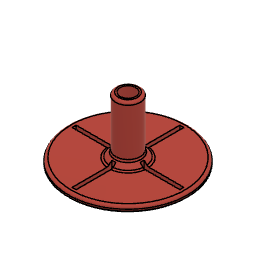
231213 drilling alignment tool 5.5 mm dia. v1 (Autodesk Fusion 360 design; units mm, degrees)
Autodesk Fusion 360 part; units mm, degrees
sketch "5.5 drilling alignment tool" plane through (0, 0, 0) normal (0, 1, 0) x (1, 0, 0)
  circle A0 centre (0, 0) radius 2.75
  circle A1 centre (0, 0) radius 4.35
  circle A2 centre (0, 0) radius 21
  line L0 (0, 0) -> (0, 30.5486) construction
  line L1 (0, 0) -> (37.4223, 0) construction
  line L2 (5, 0.7) -> (19, 0.7)
  line L3 (19, 0.7) -> (19, -0.7)
  line L4 (19, -0.7) -> (5, -0.7)
  line L5 (5, -0.7) -> (5, 0.7)
  dimension "d1" = 5.5
  dimension "d2" = 1.6
  dimension "d3" = 42
  dimension "d12" = 5
  dimension "d13" = 14
  dimension "d14" = 1.4
  constraint coincident A0.centre A1.centre
  constraint concentric A0 A2
  constraint vertical L0
  constraint perpendicular L0 L1
  constraint horizontal L2
  constraint vertical L3
  constraint horizontal L4
  constraint vertical L5
  constraint symmetric L1 L2 L4
  measures "d1" diameter of A0
  measures "d2" distance of A0 A1
  measures "d3" diameter of A2
  measures "d12" distance of A0.centre L5
  measures "d13" distance of L3 L5
  measures "d14" distance of L2 L4
extrude "Extrude1" add sketch "5.5 drilling alignment tool" along normal blind 22 contours A1
extrude "Extrude2" add sketch "5.5 drilling alignment tool" along normal blind 2 contours A2 | L2 L3 L4 L5
chamfer "Chamfer1" distance 2 angle 45 1 edges at (-4.0556, 2, 1.573)
fillet "Fillet1" radius 1 3 faces at (4.3284, 10, 0.4331) (-3.5435, 2.6667, 4.4434) (16.0385, 2, 1.0433)
chamfer "Chamfer2" distance 0.4 angle 45 1 edges at (-19.5789, 0, 7.5939)
extrude "Extrude3" cut sketch "5.5 drilling alignment tool" along normal blind 4 contours L2 L3 L4 L5
pattern_circular "C-Pattern1" count 4 over 360 about axis through (0, 1.75, 0) along (0, 1, 0) of "Extrude3"
named bodies: "5.5 drilling alignment tool"
